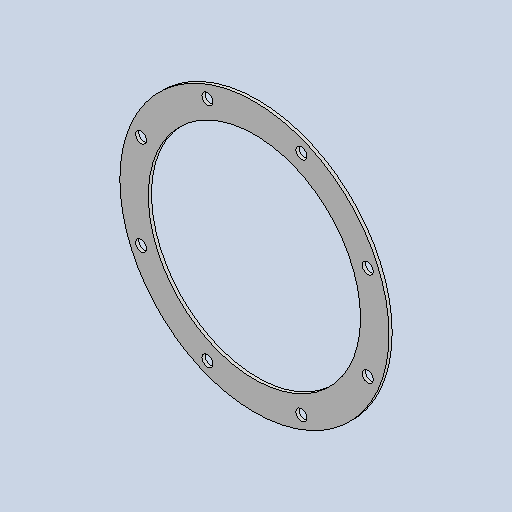
# Autodesk Inventor part: DMF 2.1 01 45 Gear ring 5_CPY1
Saved by Autodesk Inventor 2026.2 (Build 302298010, 298A)
## iProperties
Created: 2024-04-30
Part Number: DMF 2.1 01 45 Gear ring 5_CPY1
Material: Generic
Document SubType Name: Sheet Metal
Designer: admin
Stock Number: Барабан_Сектор_Усилителя
Density: 1 g/cm^3
Flat Pattern Width: 17 cm
Flat Pattern Length: 17 cm
Flat Pattern Area: 289 cm^2
Sheet Metal Rule: Default
Sheet Metal Width: 170,000 mm
Sheet Metal Length: 170,000 mm
Sheet Metal Area: 28900,000 mm^2
Appearance: Default
Mass: 16.575 g
Surface Area: 188.37 cm^2
Volume: 16.575 cm^3
Author: pokla
Autodesk Inventor part; units mm, degrees
ref_plane "YZ Plane" through (0, 0, 0) normal (1, 0, 0) x (0, 1, 0)
ref_plane "XZ Plane" through (0, 0, 0) normal (0, 1, 0) x (-1, 0, 0)
ref_plane "XY Plane" through (0, 0, 0) normal (0, 0, 1) x (1, 0, 0)
sketch "Sketch1" plane through (0, 0, 0) normal (0, 0, 1) x (1, 0, 0)
  circle A0 centre (0, 0) radius 67
  circle A1 centre (0, 0) radius 85
  line L0 (0, 0) -> (0, 67) construction
  line L1 (0, 0) -> (-85, 0) construction
  circle A2 centre (29.658, 71.6007) radius 3.5
  line L2 (29.658, 71.6007) -> (0, 0) construction
  circle A3 centre (0, 0) radius 77.5 construction
  circle A4 centre (-29.658, 71.6007) radius 3.5
  circle A5 centre (-71.6007, 29.658) radius 3.5
  circle A6 centre (-71.6007, -29.658) radius 3.5
  circle A7 centre (-29.658, -71.6007) radius 3.5
  circle A8 centre (29.658, -71.6007) radius 3.5
  circle A9 centre (71.6007, -29.658) radius 3.5
  circle A10 centre (71.6007, 29.658) radius 3.5
  point P0 (0, -85)
  dimension "d32" = 134
  dimension "d97" = 155
  dimension "d31" = 170
  dimension "d95" = 7
  dimension "d96" = 22.5
  dimension "d100" = 360
  measures "d31" diameter of A1
  measures "d95" diameter of A2
  measures "d96" angle of L2 L0
extrude "Plate4" add sketch "Sketch1" along normal blind 2
sketch "Sketch5" plane through (0, 0, 2) normal (0, 0, 1) x (1, 0, 0)
  line L0 (-1.6, -169) -> (1.6, -169)
  line L1 (1.6, -169) -> (1.6, -209)
  line L2 (1.6, -209) -> (-1.6, -209)
  line L3 (-1.6, -209) -> (-1.6, -169)
  line L4 (-207, -40) -> (-167, -40)
  line L5 (-167, -40) -> (-167, -43.2)
  line L6 (-167, -43.2) -> (-207, -43.2)
  line L7 (-207, -43.2) -> (-207, -40)
  line L8 (0, 0) -> (0, -169)
  line L9 (167, -40) -> (207, -40)
  line L10 (207, -40) -> (207, -43.2)
  line L11 (207, -43.2) -> (167, -43.2)
  line L12 (167, -43.2) -> (167, -40)
  dimension "d74" = 3.2
  dimension "d75" = 40
  dimension "d76" = 40
  dimension "d77" = 40
  dimension "d78" = 167
  dimension "d79" = 169
  constraints: 26 end point, 6 parallel, 3 equal length, 3 horizontal, 3 perpendicular, 1 collinear, 1 midpoint, 1 vertical, 1 other
  measures "d74" distance of L0.start L0.end
  measures "d75" distance of L0.end L1.end
  measures "d76" distance of L4.start L4.end
  measures "d77" distance from line of L8.start L4
  measures "d78" distance between parallel lines of L8 L5
  measures "d79" distance from line of L0 L8.start
feature "Mark1" [suppressed]
equation "\"d63\" = Thickness"
equation "\"BendRadius\" = Thickness"
equation "\"BendReliefWidth\" = Thickness"
equation "\"BendReliefDepth\" = 0.5 * Thickness"
equation "\"CornerReliefSize\" = 4 * Thickness"
equation "\"MinimumRemnant\" = 2 * Thickness"
equation "\"TransitionRadius\" = BendRadius"
equation "\"JacobiRadiusSize\" = BendRadius"
equation "\"GapSize\" = Thickness"
equation "\"Thickness\" = 2"
body "Solid3"
